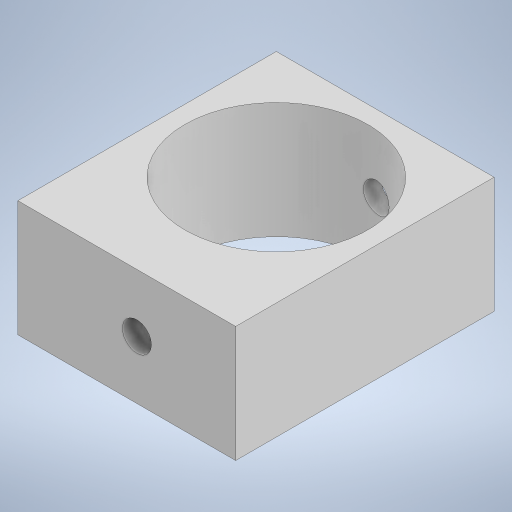
# Autodesk Inventor part: welco mount v04
Saved by Autodesk Inventor 2023 (Build 270158000, 158)
## iProperties
Created: 2024-07-10
Part Number: welco mount v04
Material: Generic
Document SubType Name: Modeling
Designer: Akramilab
Density: 1 g/cm^3
Appearance: Default
Author: Akramilab
Autodesk Inventor part; units mm, degrees
ref_plane "YZ Plane" through (0, 0, 0) normal (1, 0, 0) x (0, 1, 0)
ref_plane "XZ Plane" through (0, 0, 0) normal (0, 1, 0) x (-1, 0, 0)
ref_plane "XY Plane" through (0, 0, 0) normal (0, 0, 1) x (1, 0, 0)
sketch "Sketch1" plane through (0, 0, 0) normal (0, 1, 0) x (-1, 0, 0)
  line L0 (0, 0) -> (-37.5, 0)
  line L1 (-37.5, 0) -> (-37.5, 37.5)
  line L2 (-37.5, 37.5) -> (0, 37.5)
  line L3 (0, 37.5) -> (0, 0)
  circle A0 centre (-18.75, 18.75) radius 15.75
  point P0 (-18.75, 0)
  dimension "d0" = 37.5
  dimension "d1" = 37.5
  dimension "d2" = 18.75
  dimension "d3" = 18.75
  dimension "d4" = 31.5
  constraints: 8 end point, 2 parallel, 1 centre point, 1 coincident, 1 horizontal, 1 midpoint, 1 perpendicular
  measures "d0" distance of L1.end L2.end
  measures "d1" distance of L0.end L1.end
  measures "d2" distance of point (-18.75, 0) point (-18.75, 18.75)
  measures "d3" distance from line of L3 point (-18.75, 18.75)
  measures "d4" diameter of A0
extrude "Extrusion1" add sketch "Sketch1" against normal blind 20
sketch "Sketch3" plane through (0, 0, 37.5) normal (0, 0, 1) x (1, 0, 0)
  circle A0 centre (20.5, -10) radius 4.5
  point P0 (0, 0)
  dimension "d8" = 9
  constraints: 1 centre point, 1 coincident
  measures "d8" diameter of A0
extrude "Extrusion2" cut sketch "Sketch3" against normal blind 5
sketch "Sketch4" plane through (37.5, 0, 0) normal (0, 0, -1) x (-1, 0, 0)
  circle A0 centre (17, -10) radius 4.5 projected
  circle A1 centre (17, -10) radius 2.5
  point P0 (37.5, 0)
  dimension "d11" = 5
  constraints: 1 centre point, 1 coincident
  measures "d11" diameter of A1
extrude "Extrusion3" cut sketch "Sketch4" against normal blind 5 contours A1
sketch "Sketch5" plane through (0, 0, 37.5) normal (0, 0, 1) x (1, 0, 0)
  line L0 (37.5, 0) -> (0, 0) projected
  line L1 (0, -20) -> (37.5, -20) projected
  line L2 (0, 0) -> (37.5, 0)
  line L3 (37.5, 0) -> (37.5, -20)
  line L4 (37.5, -20) -> (0, -20)
  line L5 (0, -20) -> (0, 0)
  line L6 (0, 0) -> (0, -20) projected
  line L7 (0, 0) -> (37.5, 0)
  line L8 (37.5, 0) -> (37.5, -20)
  line L9 (37.5, -20) -> (0, -20)
  line L10 (0, -20) -> (0, 0)
  circle A0 centre (20.5, -10) radius 4.5
  constraints: 16 end point, 4 parallel, 2 horizontal, 2 perpendicular, 1 centre point
extrude "Extrusion4" add sketch "Sketch5" along normal blind 2
sketch "Sketch6" plane through (0, 0, 39.5) normal (0, 0, 1) x (1, 0, 0)
  line L0 (0, 0) -> (0, -20) projected
  line L1 (0, -20) -> (37.5, -20) projected
  line L2 (0, 0) -> (37.5, 0)
  line L3 (37.5, 0) -> (37.5, -20)
  line L4 (37.5, -20) -> (0, -20)
  line L5 (0, -20) -> (0, 0)
  circle A0 centre (20.5, -10) radius 2.5
  constraints: 8 end point, 2 parallel, 1 centre point, 1 horizontal, 1 perpendicular
extrude "Extrusion5" add sketch "Sketch6" along normal blind 5
equation "\"d0\" = d1"
equation "\"d2\" = 0.5 * d1"
equation "\"d3\" = 0.5 * d0"
body "Solid1"
